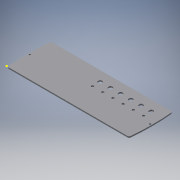
# Autodesk Inventor part: Frontplatte Apra Xdream 418
Saved by Autodesk Inventor 2018 (Build 220112000, 112)
## iProperties
Created: 2011-10-18
Part Number: Frontplatte Apra Xdream 418
Document SubType Name: Modeling
Designer: Huethe
Mass: 51.0801 g
Surface Area: 425.217 cm^2
Volume: 51.0801 cm^3
Density: 1 g/cm^3
Material: Allgemein
Appearance: Vorgabe
Author: Huethe
Autodesk Inventor part; units mm, degrees
ref_plane "YZ Plane" through (0, 0, 0) normal (1, 0, 0) x (0, 1, 0)
ref_plane "XZ Plane" through (0, 0, 0) normal (0, 1, 0) x (-1, 0, 0)
ref_plane "XY Plane" through (0, 0, 0) normal (0, 0, 1) x (1, 0, 0)
sketch "Skizze1" plane through (0, 0, 0) normal (0, 0, 1) x (1, 0, 0)
  line L0 (0, 0) -> (242, 0)
  line L1 (242, 0) -> (242, 85)
  line L2 (242, 85) -> (0, 85)
  line L3 (0, 85) -> (0, 0)
  line L4 (242, 42.5) -> (842, 42.5)
  line L5 (0, 42.5) -> (-937, 42.5)
  arc A0 (240, 0) -> (240, 85) centre (-210.5625, 42.5) ccw
  arc A1 (2, 85) -> (2, 0) centre (452.5625, 42.5) ccw
  dimension "d0" = 85
  dimension "d1" = 242
  dimension "d2" = 2
  dimension "d3" = 2
  dimension "d4" = 2
  dimension "d7" = 452.5625
  dimension "d8" = 452.5625
  constraints: 12 end point, 6 point on line, 4 point on circle, 2 centre point, 2 midpoint, 2 parallel, 2 tangent, 1 collinear, 1 horizontal, 1 perpendicular
  measures "d0" distance between parallel lines of L0 L2
  measures "d1" distance between parallel lines of L1 L3
  measures "d2" distance from line of L3 A1.start
  measures "d3" distance from line of A1.end L3
  measures "d4" distance from line of L1 A0.end
  measures "d7" radius of A0
  measures "d8" radius of A1
extrude "Extrusion1" add sketch "Skizze1" against normal blind 2.5 contours A1 L2 A0 L0
sketch "Skizze2" plane through (0, 0, 0) normal (0, 0, 1) x (1, 0, 0)
  line L0 (2, 0) -> (240, 0) projected
  line L1 (240, 85) -> (2, 85) projected
  line L2 (121, 0) -> (121, 85)
  point P0 (0, 0)
  point P1 (3.1, 42.5)
  point P2 (238.9, 42.5)
  dimension "d11" = 42.5
  dimension "d12" = 42.5
  dimension "d13" = 235.8
  dimension "d14" = 117.9
  dimension "d15" = 117.9
  constraints: 2 end point, 2 midpoint
  measures "d11" distance from line of L0 point (3.1, 42.5)
  measures "d12" distance from line of L0 point (238.9, 42.5)
  measures "d13" distance of point (238.9, 42.5) point (3.1, 42.5)
  measures "d14" distance from line of L2 point (3.1, 42.5)
  measures "d15" distance from line of L2 point (238.9, 42.5)
hole "Bohrung1" at (3.1, 42.5, 0) at (238.9, 42.5, 0) direction (0, 0, -1) diameter 3.3 depth 8 tip angle 118
sketch "Skizze3" plane through (0, 0, 0) normal (0, 0, 1) x (1, 0, 0)
  line L0 (2, 0) -> (240, 0) projected
  line L1 (240, 85) -> (2, 85) projected
  arc A0 (2, 85) -> (2, 0) centre (452.5625, 42.5) ccw projected
  line L2 (8.1386, 91.5936) -> (-1.2688, 78.1585)
  line L3 (-1.2688, 78.1585) -> (-1.2688, 91.5936)
  line L4 (-1.2688, 91.5936) -> (8.1386, 91.5936)
  line L5 (-1.7926, 7.5896) -> (9.0296, -7.8661)
  line L6 (9.0296, -7.8661) -> (-1.7926, -7.8661)
  line L7 (-1.7926, -7.8661) -> (-1.7926, 7.5896)
  line L8 (121, 0) -> (121, 85)
  line L9 (233.8614, 91.5936) -> (243.2688, 78.1585)
  line L10 (243.2688, 78.1585) -> (243.2688, 91.5936)
  line L11 (243.2688, 91.5936) -> (233.8614, 91.5936)
  line L12 (243.7926, 7.5896) -> (232.9704, -7.8661)
  line L13 (232.9704, -7.8661) -> (243.7926, -7.8661)
  line L14 (243.7926, -7.8661) -> (243.7926, 7.5896)
  point P0 (0, 0)
  point P1 (1.7712, 82.5)
  point P2 (1.7712, 2.5)
  point P3 (242, 0)
  point P4 (240.2288, 82.5)
  point P5 (240.2288, 2.5)
  dimension "d23" = 55
  dimension "d24" = 55
  dimension "d25" = 2.5
  dimension "d26" = 2.5
  constraints: 26 end point, 9 symmetric about line, 4 point on line, 3 perpendicular, 2 midpoint, 2 point on circle, 1 parallel
  measures "d23" angle of L2 L4
  measures "d24" angle of L6 L5
  measures "d25" distance from line of L0 point (1.771, 2.5)
  measures "d26" distance from line of L1 point (1.771, 82.5)
extrude "Extrusion2" cut sketch "Skizze3" against normal blind 5 contours A0 L5 L0 | L0 L5 L6 L7 A0 | L9 L11 L10 | L12 L14 L13 | L2 L3 L4 L1 A0 | A0 L1 L2
sketch "Sketch7" plane through (0, 0, 0) normal (0, 0, 1) x (1, 0, 0)
  point P0 (0, 0)
sketch "Sketch9" plane through (0, 0, -2.5) normal (0, 0, -1) x (-1, 0, 0)
  line L0 (-238.4783, 85) -> (-3.5217, 85) projected
  line L1 (-214.9283, 63.0506) -> (-222.0283, 63.0506) construction
  line L2 (-222.0283, 63.0506) -> (-222.0283, 66.9494)
  line L3 (-222.0283, 66.9494) -> (-214.9283, 66.9494) construction
  line L4 (-214.9283, 66.9494) -> (-214.9283, 63.0506)
  line L5 (-214.9283, 63.0506) -> (-222.0283, 66.9494) construction
  line L6 (-222.0283, 63.0506) -> (-214.9283, 66.9494) construction
  arc A0 (-222.0283, 63.0506) -> (-214.9283, 63.0506) centre (-218.4783, 65) ccw
  arc A1 (-214.9283, 66.9494) -> (-222.0283, 66.9494) centre (-218.4783, 65) ccw
  line L7 (-194.9283, 63.0506) -> (-202.0283, 63.0506) construction
  line L8 (-202.0283, 63.0506) -> (-202.0283, 66.9494)
  line L9 (-202.0283, 66.9494) -> (-194.9283, 66.9494) construction
  line L10 (-194.9283, 66.9494) -> (-194.9283, 63.0506)
  line L11 (-194.9283, 63.0506) -> (-202.0283, 66.9494) construction
  line L12 (-202.0283, 63.0506) -> (-194.9283, 66.9494) construction
  arc A2 (-202.0283, 63.0506) -> (-194.9283, 63.0506) centre (-198.4783, 65) ccw
  arc A3 (-194.9283, 66.9494) -> (-202.0283, 66.9494) centre (-198.4783, 65) ccw
  line L13 (-174.9283, 63.0506) -> (-182.0283, 63.0506) construction
  line L14 (-182.0283, 63.0506) -> (-182.0283, 66.9494)
  line L15 (-182.0283, 66.9494) -> (-174.9283, 66.9494) construction
  line L16 (-174.9283, 66.9494) -> (-174.9283, 63.0506)
  line L17 (-174.9283, 63.0506) -> (-182.0283, 66.9494) construction
  line L18 (-182.0283, 63.0506) -> (-174.9283, 66.9494) construction
  arc A4 (-182.0283, 63.0506) -> (-174.9283, 63.0506) centre (-178.4783, 65) ccw
  arc A5 (-174.9283, 66.9494) -> (-182.0283, 66.9494) centre (-178.4783, 65) ccw
  line L19 (-154.9283, 63.0506) -> (-162.0283, 63.0506) construction
  line L20 (-162.0283, 63.0506) -> (-162.0283, 66.9494)
  line L21 (-162.0283, 66.9494) -> (-154.9283, 66.9494) construction
  line L22 (-154.9283, 66.9494) -> (-154.9283, 63.0506)
  line L23 (-154.9283, 63.0506) -> (-162.0283, 66.9494) construction
  line L24 (-162.0283, 63.0506) -> (-154.9283, 66.9494) construction
  arc A6 (-162.0283, 63.0506) -> (-154.9283, 63.0506) centre (-158.4783, 65) ccw
  arc A7 (-154.9283, 66.9494) -> (-162.0283, 66.9494) centre (-158.4783, 65) ccw
  line L25 (-134.9283, 63.0506) -> (-142.0283, 63.0506) construction
  line L26 (-142.0283, 63.0506) -> (-142.0283, 66.9494)
  line L27 (-142.0283, 66.9494) -> (-134.9283, 66.9494) construction
  line L28 (-134.9283, 66.9494) -> (-134.9283, 63.0506)
  line L29 (-134.9283, 63.0506) -> (-142.0283, 66.9494) construction
  line L30 (-142.0283, 63.0506) -> (-134.9283, 66.9494) construction
  arc A8 (-142.0283, 63.0506) -> (-134.9283, 63.0506) centre (-138.4783, 65) ccw
  arc A9 (-134.9283, 66.9494) -> (-142.0283, 66.9494) centre (-138.4783, 65) ccw
  line L31 (-114.9283, 63.0506) -> (-122.0283, 63.0506) construction
  line L32 (-122.0283, 63.0506) -> (-122.0283, 66.9494)
  line L33 (-122.0283, 66.9494) -> (-114.9283, 66.9494) construction
  line L34 (-114.9283, 66.9494) -> (-114.9283, 63.0506)
  line L35 (-114.9283, 63.0506) -> (-122.0283, 66.9494) construction
  line L36 (-122.0283, 63.0506) -> (-114.9283, 66.9494) construction
  arc A10 (-122.0283, 63.0506) -> (-114.9283, 63.0506) centre (-118.4783, 65) ccw
  arc A11 (-114.9283, 66.9494) -> (-122.0283, 66.9494) centre (-118.4783, 65) ccw
  circle A12 centre (-218.4783, 50) radius 2.4
  circle A13 centre (-198.4783, 50) radius 2.4
  circle A14 centre (-178.4783, 50) radius 2.4
  circle A15 centre (-158.4783, 50) radius 2.4
  circle A16 centre (-138.4783, 50) radius 2.4
  circle A17 centre (-118.4783, 50) radius 2.4
  point P0 (0, 0)
  dimension "d97" = 20
  dimension "d98" = 20
  dimension "d99" = 7.1
  dimension "d100" = 4.05
  dimension "d103" = 20
  dimension "d108" = 15
  dimension "d109" = 4.8
  dimension "d112" = 20
  constraints: 72 end point, 24 point on circle, 18 centre point, 13 midpoint, 3 horizontal, 2 parallel, 1 perpendicular, 1 vertical alignment, 75 other
  measures "d97" distance from line of L0 A0.centre
  measures "d98" horizontal distance of A0.centre L0.start
  measures "d99" distance of L2.end L3.end
  measures "d100" radius of A0
  measures "d103" distance of A0.centre A2.centre
  measures "d108" distance of A12.centre A0.centre
  measures "d109" diameter of A12
  measures "d112" distance of A12.centre A13.centre
extrude "Extrusion6" cut sketch "Sketch9" against normal blind 3
